Autodesk Fusion 360 part; units mm, degrees
note: some values were not read from the file. Set by a fixed rule: which face or edge a step refers to.
(part 2 of 2)
sketch "Sketch7" plane through (71, 0, 0) normal (1, 0, 0) x (0, 1, 0)
  line L0 (-31, -12) -> (369, -12)
  line L1 (369, -12) -> (348.4062, 44.7862)
  line L2 (348.4062, 44.7862) -> (327.7275, 73.6318)
  line L3 (327.7275, 73.6318) -> (172.6327, 98)
  line L4 (172.6327, 98) -> (-31, 98)
  line L5 (-31, 98) -> (-31, -12)
  line L6 (324.7064, 35.6875) -> (319.5665, 44.4255)
  arc A0 (328.6078, 48.7783) -> (319.5665, 44.4255) centre (321.9697, 51) ccw
  line L7 (328.6078, 48.7783) -> (333.3258, 40.7577)
  arc A1 (338.2936, 32.3125) -> (333.3258, 40.7577) centre (331.5, 34) ccw
  line L8 (338.2936, 32.3125) -> (343.3258, 23.7577)
  arc A2 (348.3189, 15.4181) -> (343.3258, 23.7577) centre (341.5, 17) ccw
  line L9 (348.3189, 15.4181) -> (353.8077, 6.4122)
  arc A3 (346.101, -5) -> (353.8077, 6.4122) centre (351, 0) ccw
  line L10 (346.101, -5) -> (336.399, -5)
  arc A4 (326.601, -5) -> (336.399, -5) centre (331.5, 0) ccw
  line L11 (326.601, -5) -> (316.899, -5)
  arc A5 (310.0903, 6.7345) -> (316.899, -5) centre (312, 0) ccw
  line L12 (310.0903, 6.7345) -> (315.1571, 15.5255)
  arc A6 (319.8454, 23.6602) -> (315.1571, 15.5255) centre (322, 17) ccw
  line L13 (319.8454, 23.6602) -> (324.7456, 32.1622)
  arc A7 (324.7064, 35.6875) -> (324.7456, 32.1622) centre (331.5, 34) ccw
  line L14 (66.4689, 57.708) -> (71.277, 66.0503)
  arc A8 (76.3168, 74.7946) -> (71.277, 66.0503) centre (78, 68) ccw
  line L15 (76.3168, 74.7946) -> (81.1914, 83.2523)
  arc A9 (89.8554, 78.2588) -> (81.1914, 83.2523) centre (87.9697, 85) ccw
  line L16 (89.8554, 78.2588) -> (84.829, 69.5378)
  arc A10 (80.0928, 61.3202) -> (84.829, 69.5378) centre (78, 68) ccw
  line L17 (80.0928, 61.3202) -> (75.2176, 52.8615)
  arc A11 (75.1078, 48.7783) -> (75.2176, 52.8615) centre (68.4697, 51) ccw
  line L18 (75.1078, 48.7783) -> (79.8258, 40.7577)
  arc A12 (84.7936, 32.3125) -> (79.8258, 40.7577) centre (78, 34) ccw
  line L19 (84.7936, 32.3125) -> (89.8258, 23.7577)
  arc A13 (89.6246, 10.1911) -> (89.8258, 23.7577) centre (88, 17) ccw
  line L20 (89.6246, 10.1911) -> (84.7721, 1.7718)
  arc A14 (71.3471, 2.177) -> (84.7721, 1.7718) centre (78, 0) ccw
  line L21 (71.3471, 2.177) -> (66.6451, 10.2502)
  arc A15 (66.3454, 23.6602) -> (66.6451, 10.2502) centre (68.5, 17) ccw
  line L22 (66.3454, 23.6602) -> (71.2456, 32.1622)
  arc A16 (71.2064, 35.6875) -> (71.2456, 32.1622) centre (78, 34) ccw
  line L23 (71.2064, 35.6875) -> (66.0665, 44.4255)
  arc A17 (66.4689, 57.708) -> (66.0665, 44.4255) centre (68.4697, 51) ccw
  line L24 (32.0797, 69.053) -> (26.3996, 78.7092)
  arc A18 (35.9118, 82.2615) -> (26.3996, 78.7092) centre (29.4697, 85) ccw
  line L25 (35.9118, 82.2615) -> (40.2494, 74.8876)
  arc A19 (41.0928, 61.3202) -> (40.2494, 74.8876) centre (39, 68) ccw
  line L26 (41.0928, 61.3202) -> (36.2176, 52.8615)
  arc A20 (36.1078, 48.7783) -> (36.2176, 52.8615) centre (29.4697, 51) ccw
  line L27 (36.1078, 48.7783) -> (40.8258, 40.7577)
  arc A21 (40.9765, 27.2848) -> (40.8258, 40.7577) centre (39, 34) ccw
  line L28 (40.9765, 27.2848) -> (36.2059, 19.0076)
  arc A22 (36.3189, 15.4181) -> (36.2059, 19.0076) centre (29.5, 17) ccw
  line L29 (36.3189, 15.4181) -> (41.8077, 6.4122)
  arc A23 (32.3471, 2.177) -> (41.8077, 6.4122) centre (39, 0) ccw
  line L30 (32.3471, 2.177) -> (27.6451, 10.2502)
  arc A24 (22.7064, 18.6875) -> (27.6451, 10.2502) centre (29.5, 17) ccw
  line L31 (22.7064, 18.6875) -> (17.6742, 27.2423)
  arc A25 (17.7042, 40.7657) -> (17.6742, 27.2423) centre (19.5, 34) ccw
  line L32 (17.7042, 40.7657) -> (22.6625, 49.3685)
  arc A26 (27.4689, 57.708) -> (22.6625, 49.3685) centre (29.4697, 51) ccw
  line L33 (27.4689, 57.708) -> (32.277, 66.0503)
  arc A27 (32.0797, 69.053) -> (32.277, 66.0503) centre (39, 68) ccw
  line L34 (-1.6832, 74.7946) -> (3.1914, 83.2523)
  arc A28 (16.4118, 82.2615) -> (3.1914, 83.2523) centre (9.9697, 85) ccw
  line L35 (16.4118, 82.2615) -> (20.7494, 74.8876)
  arc A29 (21.5928, 61.3202) -> (20.7494, 74.8876) centre (19.5, 68) ccw
  line L36 (21.5928, 61.3202) -> (16.7176, 52.8615)
  arc A30 (11.7417, 44.228) -> (16.7176, 52.8615) centre (9.9697, 51) ccw
  line L37 (11.7417, 44.228) -> (6.8013, 35.6561)
  arc A31 (6.7936, 32.3125) -> (6.8013, 35.6561) centre (0, 34) ccw
  line L38 (6.7936, 32.3125) -> (11.8258, 23.7577)
  arc A32 (16.8189, 15.4181) -> (11.8258, 23.7577) centre (10, 17) ccw
  line L39 (16.8189, 15.4181) -> (22.3077, 6.4122)
  arc A33 (12.8471, 2.177) -> (22.3077, 6.4122) centre (19.5, 0) ccw
  line L40 (12.8471, 2.177) -> (8.1451, 10.2502)
  arc A34 (3.2064, 18.6875) -> (8.1451, 10.2502) centre (10, 17) ccw
  line L41 (3.2064, 18.6875) -> (-1.8258, 27.2423)
  arc A35 (-1.7958, 40.7657) -> (-1.8258, 27.2423) centre (0, 34) ccw
  line L42 (-1.7958, 40.7657) -> (3.1625, 49.3685)
  arc A36 (3.0557, 52.0938) -> (3.1625, 49.3685) centre (9.9697, 51) ccw
  line L43 (3.0557, 52.0938) -> (-2.4419, 61.4397)
  arc A37 (-1.6832, 74.7946) -> (-2.4419, 61.4397) centre (0, 68) ccw
  line L44 (-21.1832, 74.7946) -> (-16.3086, 83.2523)
  arc A38 (-7.6446, 78.2588) -> (-16.3086, 83.2523) centre (-9.5303, 85) ccw
  line L45 (-7.6446, 78.2588) -> (-12.671, 69.5378)
  arc A39 (-12.873, 65.7456) -> (-12.671, 69.5378) centre (-19.5, 68) ccw
  line L46 (-12.873, 65.7456) -> (-8.2469, 57.8813)
  arc A40 (-7.7583, 44.228) -> (-8.2469, 57.8813) centre (-9.5303, 51) ccw
  line L47 (-7.7583, 44.228) -> (-12.6987, 35.6561)
  arc A41 (-12.7064, 32.3125) -> (-12.6987, 35.6561) centre (-19.5, 34) ccw
  line L48 (-12.7064, 32.3125) -> (-7.6742, 23.7577)
  arc A42 (-2.6811, 15.4181) -> (-7.6742, 23.7577) centre (-9.5, 17) ccw
  line L49 (-2.6811, 15.4181) -> (2.8077, 6.4122)
  arc A43 (-4.899, -5) -> (2.8077, 6.4122) centre (0, 0) ccw
  line L50 (-4.899, -5) -> (-14.601, -5)
  arc A44 (-21.4097, 6.7345) -> (-14.601, -5) centre (-19.5, 0) ccw
  line L51 (-21.4097, 6.7345) -> (-16.3429, 15.5255)
  arc A45 (-16.2936, 18.6875) -> (-16.3429, 15.5255) centre (-9.5, 17) ccw
  line L52 (-16.2936, 18.6875) -> (-21.3258, 27.2423)
  arc A46 (-21.2958, 40.7657) -> (-21.3258, 27.2423) centre (-19.5, 34) ccw
  line L53 (-21.2958, 40.7657) -> (-16.3375, 49.3685)
  arc A47 (-16.4443, 52.0938) -> (-16.3375, 49.3685) centre (-9.5303, 51) ccw
  line L54 (-16.4443, 52.0938) -> (-21.9419, 61.4397)
  arc A48 (-21.1832, 74.7946) -> (-21.9419, 61.4397) centre (-19.5, 68) ccw
  line L55 (193.3168, 74.7946) -> (194.7952, 77.3597)
  line L56 (194.7952, 77.3597) -> (196.2494, 74.8876)
  arc A49 (201.627, 65.7456) -> (196.2494, 74.8876) centre (195, 68) ccw
  line L57 (201.627, 65.7456) -> (206.2531, 57.8813)
  arc A50 (206.7417, 44.228) -> (206.2531, 57.8813) centre (204.9697, 51) ccw
  line L58 (206.7417, 44.228) -> (201.8013, 35.6561)
  arc A51 (201.7936, 32.3125) -> (201.8013, 35.6561) centre (195, 34) ccw
  line L59 (201.7936, 32.3125) -> (206.8258, 23.7577)
  arc A52 (206.6246, 10.1911) -> (206.8258, 23.7577) centre (205, 17) ccw
  line L60 (206.6246, 10.1911) -> (201.7721, 1.7718)
  arc A53 (188.3471, 2.177) -> (201.7721, 1.7718) centre (195, 0) ccw
  line L61 (188.3471, 2.177) -> (183.6451, 10.2502)
  arc A54 (183.3454, 23.6602) -> (183.6451, 10.2502) centre (185.5, 17) ccw
  line L62 (183.3454, 23.6602) -> (188.2456, 32.1622)
  arc A55 (188.2064, 35.6875) -> (188.2456, 32.1622) centre (195, 34) ccw
  line L63 (188.2064, 35.6875) -> (183.0665, 44.4255)
  arc A56 (183.4689, 57.708) -> (183.0665, 44.4255) centre (185.4697, 51) ccw
  line L64 (183.4689, 57.708) -> (188.277, 66.0503)
  arc A57 (193.3168, 74.7946) -> (188.277, 66.0503) centre (195, 68) ccw
  line L65 (55.8189, 15.4181) -> (61.3077, 6.4122)
  arc A58 (51.8471, 2.177) -> (61.3077, 6.4122) centre (58.5, 0) ccw
  line L66 (51.8471, 2.177) -> (47.1451, 10.2502)
  arc A59 (46.8454, 23.6602) -> (47.1451, 10.2502) centre (49, 17) ccw
  line L67 (46.8454, 23.6602) -> (51.7456, 32.1622)
  arc A60 (51.7064, 35.6875) -> (51.7456, 32.1622) centre (58.5, 34) ccw
  line L68 (51.7064, 35.6875) -> (46.5665, 44.4255)
  arc A61 (46.9689, 57.708) -> (46.5665, 44.4255) centre (48.9697, 51) ccw
  line L69 (46.9689, 57.708) -> (51.777, 66.0503)
  arc A62 (51.5797, 69.053) -> (51.777, 66.0503) centre (58.5, 68) ccw
  line L70 (51.5797, 69.053) -> (45.8996, 78.7092)
  arc A63 (53.8686, 90) -> (45.8996, 78.7092) centre (48.9697, 85) ccw
  line L71 (53.8686, 90) -> (63.5707, 90)
  arc A64 (70.3554, 78.2588) -> (63.5707, 90) centre (68.4697, 85) ccw
  line L72 (70.3554, 78.2588) -> (65.329, 69.5378)
  arc A65 (60.5928, 61.3202) -> (65.329, 69.5378) centre (58.5, 68) ccw
  line L73 (60.5928, 61.3202) -> (55.7176, 52.8615)
  arc A66 (55.6078, 48.7783) -> (55.7176, 52.8615) centre (48.9697, 51) ccw
  line L74 (55.6078, 48.7783) -> (60.3258, 40.7577)
  arc A67 (60.4765, 27.2848) -> (60.3258, 40.7577) centre (58.5, 34) ccw
  line L75 (60.4765, 27.2848) -> (55.7059, 19.0076)
  arc A68 (55.8189, 15.4181) -> (55.7059, 19.0076) centre (49, 17) ccw
  line L76 (95.8168, 74.7946) -> (100.6914, 83.2523)
  arc A69 (109.3554, 78.2588) -> (100.6914, 83.2523) centre (107.4697, 85) ccw
  line L77 (109.3554, 78.2588) -> (104.329, 69.5378)
  arc A70 (104.127, 65.7456) -> (104.329, 69.5378) centre (97.5, 68) ccw
  line L78 (104.127, 65.7456) -> (108.7531, 57.8813)
  arc A71 (109.2417, 44.228) -> (108.7531, 57.8813) centre (107.4697, 51) ccw
  line L79 (109.2417, 44.228) -> (104.3013, 35.6561)
  arc A72 (104.2936, 32.3125) -> (104.3013, 35.6561) centre (97.5, 34) ccw
  line L80 (104.2936, 32.3125) -> (109.3258, 23.7577)
  arc A73 (109.1246, 10.1911) -> (109.3258, 23.7577) centre (107.5, 17) ccw
  line L81 (109.1246, 10.1911) -> (104.2721, 1.7718)
  arc A74 (95.5903, 6.7345) -> (104.2721, 1.7718) centre (97.5, 0) ccw
  line L82 (95.5903, 6.7345) -> (100.6571, 15.5255)
  arc A75 (100.7064, 18.6875) -> (100.6571, 15.5255) centre (107.5, 17) ccw
  line L83 (100.7064, 18.6875) -> (95.6742, 27.2423)
  arc A76 (90.7064, 35.6875) -> (95.6742, 27.2423) centre (97.5, 34) ccw
  line L84 (90.7064, 35.6875) -> (85.5665, 44.4255)
  arc A77 (85.9689, 57.708) -> (85.5665, 44.4255) centre (87.9697, 51) ccw
  line L85 (85.9689, 57.708) -> (90.777, 66.0503)
  arc A78 (95.8168, 74.7946) -> (90.777, 66.0503) centre (97.5, 68) ccw
  line L86 (268.101, -5) -> (258.399, -5)
  arc A79 (251.5903, 6.7345) -> (258.399, -5) centre (253.5, 0) ccw
  line L87 (251.5903, 6.7345) -> (256.6571, 15.5255)
  arc A80 (256.7064, 18.6875) -> (256.6571, 15.5255) centre (263.5, 17) ccw
  line L88 (256.7064, 18.6875) -> (251.6742, 27.2423)
  arc A81 (246.7064, 35.6875) -> (251.6742, 27.2423) centre (253.5, 34) ccw
  line L89 (246.7064, 35.6875) -> (241.5665, 44.4255)
  arc A82 (248.8686, 56) -> (241.5665, 44.4255) centre (243.9697, 51) ccw
  line L90 (248.8686, 56) -> (258.5707, 56)
  arc A83 (270.1078, 48.7783) -> (258.5707, 56) centre (263.4697, 51) ccw
  line L91 (270.1078, 48.7783) -> (274.8258, 40.7577)
  arc A84 (274.9765, 27.2848) -> (274.8258, 40.7577) centre (273, 34) ccw
  line L92 (274.9765, 27.2848) -> (270.2059, 19.0076)
  arc A85 (270.3189, 15.4181) -> (270.2059, 19.0076) centre (263.5, 17) ccw
  line L93 (270.3189, 15.4181) -> (275.8077, 6.4122)
  arc A86 (268.101, -5) -> (275.8077, 6.4122) centre (273, 0) ccw
  line L94 (134.8168, 74.7946) -> (139.6914, 83.2523)
  arc A87 (148.3554, 78.2588) -> (139.6914, 83.2523) centre (146.4697, 85) ccw
  line L95 (148.3554, 78.2588) -> (143.329, 69.5378)
  arc A88 (143.127, 65.7456) -> (143.329, 69.5378) centre (136.5, 68) ccw
  line L96 (143.127, 65.7456) -> (147.7531, 57.8813)
  arc A89 (153.1078, 48.7783) -> (147.7531, 57.8813) centre (146.4697, 51) ccw
  line L97 (153.1078, 48.7783) -> (157.8258, 40.7577)
  arc A90 (157.9765, 27.2848) -> (157.8258, 40.7577) centre (156, 34) ccw
  line L98 (157.9765, 27.2848) -> (153.2059, 19.0076)
  arc A91 (153.3189, 15.4181) -> (153.2059, 19.0076) centre (146.5, 17) ccw
  line L99 (153.3189, 15.4181) -> (158.8077, 6.4122)
  arc A92 (149.3471, 2.177) -> (158.8077, 6.4122) centre (156, 0) ccw
  line L100 (149.3471, 2.177) -> (144.6451, 10.2502)
  arc A93 (139.7064, 18.6875) -> (144.6451, 10.2502) centre (146.5, 17) ccw
  line L101 (139.7064, 18.6875) -> (134.6742, 27.2423)
  arc A94 (134.7042, 40.7657) -> (134.6742, 27.2423) centre (136.5, 34) ccw
  line L102 (134.7042, 40.7657) -> (139.6625, 49.3685)
  arc A95 (139.5557, 52.0938) -> (139.6625, 49.3685) centre (146.4697, 51) ccw
  line L103 (139.5557, 52.0938) -> (134.0581, 61.4397)
  arc A96 (134.8168, 74.7946) -> (134.0581, 61.4397) centre (136.5, 68) ccw
  line L104 (280.8454, 23.6602) -> (285.7456, 32.1622)
  arc A97 (285.7064, 35.6875) -> (285.7456, 32.1622) centre (292.5, 34) ccw
  line L105 (285.7064, 35.6875) -> (280.5665, 44.4255)
  arc A98 (287.8686, 56) -> (280.5665, 44.4255) centre (282.9697, 51) ccw
  line L106 (287.8686, 56) -> (297.5707, 56)
  arc A99 (309.1078, 48.7783) -> (297.5707, 56) centre (302.4697, 51) ccw
  line L107 (309.1078, 48.7783) -> (313.8258, 40.7577)
  arc A100 (313.9765, 27.2848) -> (313.8258, 40.7577) centre (312, 34) ccw
  line L108 (313.9765, 27.2848) -> (309.2059, 19.0076)
  arc A101 (304.1246, 10.1911) -> (309.2059, 19.0076) centre (302.5, 17) ccw
  line L109 (304.1246, 10.1911) -> (299.2721, 1.7718)
  arc A102 (285.8471, 2.177) -> (299.2721, 1.7718) centre (292.5, 0) ccw
  line L110 (285.8471, 2.177) -> (281.1451, 10.2502)
  arc A103 (280.8454, 23.6602) -> (281.1451, 10.2502) centre (283, 17) ccw
  line L111 (172.8189, 15.4181) -> (178.3077, 6.4122)
  arc A104 (168.8471, 2.177) -> (178.3077, 6.4122) centre (175.5, 0) ccw
  line L112 (168.8471, 2.177) -> (164.1451, 10.2502)
  arc A105 (163.8454, 23.6602) -> (164.1451, 10.2502) centre (166, 17) ccw
  line L113 (163.8454, 23.6602) -> (168.7456, 32.1622)
  arc A106 (168.7064, 35.6875) -> (168.7456, 32.1622) centre (175.5, 34) ccw
  line L114 (168.7064, 35.6875) -> (163.5665, 44.4255)
  arc A107 (159.0557, 52.0938) -> (163.5665, 44.4255) centre (165.9697, 51) ccw
  line L115 (159.0557, 52.0938) -> (153.5581, 61.4397)
  arc A108 (154.3168, 74.7946) -> (153.5581, 61.4397) centre (156, 68) ccw
  line L116 (154.3168, 74.7946) -> (159.1914, 83.2523)
  arc A109 (172.4118, 82.2615) -> (159.1914, 83.2523) centre (165.9697, 85) ccw
  line L117 (172.4118, 82.2615) -> (176.7494, 74.8876)
  arc A110 (177.5928, 61.3202) -> (176.7494, 74.8876) centre (175.5, 68) ccw
  line L118 (177.5928, 61.3202) -> (172.7176, 52.8615)
  arc A111 (172.6078, 48.7783) -> (172.7176, 52.8615) centre (165.9697, 51) ccw
  line L119 (172.6078, 48.7783) -> (177.3258, 40.7577)
  arc A112 (177.4765, 27.2848) -> (177.3258, 40.7577) centre (175.5, 34) ccw
  line L120 (177.4765, 27.2848) -> (172.7059, 19.0076)
  arc A113 (172.8189, 15.4181) -> (172.7059, 19.0076) centre (166, 17) ccw
  line L121 (115.3168, 74.7946) -> (120.1914, 83.2523)
  arc A114 (128.8554, 78.2588) -> (120.1914, 83.2523) centre (126.9697, 85) ccw
  line L122 (128.8554, 78.2588) -> (123.829, 69.5378)
  arc A115 (123.627, 65.7456) -> (123.829, 69.5378) centre (117, 68) ccw
  line L123 (123.627, 65.7456) -> (128.2531, 57.8813)
  arc A116 (128.7417, 44.228) -> (128.2531, 57.8813) centre (126.9697, 51) ccw
  line L124 (128.7417, 44.228) -> (123.8013, 35.6561)
  arc A117 (123.7936, 32.3125) -> (123.8013, 35.6561) centre (117, 34) ccw
  line L125 (123.7936, 32.3125) -> (128.8258, 23.7577)
  arc A118 (133.8189, 15.4181) -> (128.8258, 23.7577) centre (127, 17) ccw
  line L126 (133.8189, 15.4181) -> (139.3077, 6.4122)
  arc A119 (131.601, -5) -> (139.3077, 6.4122) centre (136.5, 0) ccw
  line L127 (131.601, -5) -> (121.899, -5)
  arc A120 (115.0903, 6.7345) -> (121.899, -5) centre (117, 0) ccw
  line L128 (115.0903, 6.7345) -> (120.1571, 15.5255)
  arc A121 (120.2064, 18.6875) -> (120.1571, 15.5255) centre (127, 17) ccw
  line L129 (120.2064, 18.6875) -> (115.1742, 27.2423)
  arc A122 (115.2042, 40.7657) -> (115.1742, 27.2423) centre (117, 34) ccw
  line L130 (115.2042, 40.7657) -> (120.1625, 49.3685)
  arc A123 (120.0557, 52.0938) -> (120.1625, 49.3685) centre (126.9697, 51) ccw
  line L131 (120.0557, 52.0938) -> (114.5581, 61.4397)
  arc A124 (115.3168, 74.7946) -> (114.5581, 61.4397) centre (117, 68) ccw
  line L132 (212.7042, 40.7657) -> (217.6625, 49.3685)
  arc A125 (231.1078, 48.7783) -> (217.6625, 49.3685) centre (224.4697, 51) ccw
  line L133 (231.1078, 48.7783) -> (235.8258, 40.7577)
  arc A126 (240.7936, 32.3125) -> (235.8258, 40.7577) centre (234, 34) ccw
  line L134 (240.7936, 32.3125) -> (245.8258, 23.7577)
  arc A127 (245.6246, 10.1911) -> (245.8258, 23.7577) centre (244, 17) ccw
  line L135 (245.6246, 10.1911) -> (240.7721, 1.7718)
  arc A128 (229.101, -5) -> (240.7721, 1.7718) centre (234, 0) ccw
  line L136 (229.101, -5) -> (219.399, -5)
  arc A129 (212.5903, 6.7345) -> (219.399, -5) centre (214.5, 0) ccw
  line L137 (212.5903, 6.7345) -> (217.6571, 15.5255)
  arc A130 (217.7064, 18.6875) -> (217.6571, 15.5255) centre (224.5, 17) ccw
  line L138 (217.7064, 18.6875) -> (212.6742, 27.2423)
  arc A131 (212.7042, 40.7657) -> (212.6742, 27.2423) centre (214.5, 34) ccw
  line L139 (-9.5303, 85) -> (165.9697, 85) construction
  line L140 (-18.3947, 90) -> (350, 90)
  line L141 (-45, 80) -> (350, 80)
  line L142 (-45, 63) -> (350, 63)
  line L143 (-18.3947, 73) -> (350, 73)
  line L144 (-45, 46) -> (350, 46)
  line L145 (-18.3947, 56) -> (350, 56)
  line L146 (-45, 29) -> (350, 29)
  line L147 (-18.3947, 39) -> (350, 39)
  line L148 (-45, 12) -> (350, 12)
  line L149 (-18.3947, 22) -> (350, 22)
  line L150 (-45, -5) -> (350, -5)
  line L151 (-18.3947, 5) -> (350, 5)
  line L152 (-12.0046, 90) -> (-12.0046, 102)
  line L153 (-7.9736, 90) -> (-7.9736, 102)
  line L154 (-12.0046, 96) -> (-7.9736, 96)
  line L155 (321.9697, 58) -> (317.9396, 75.1697)
  line L156 (317.0707, 56) -> (312.3656, 76.0454)
  line L157 (313.4417, 71.4611) -> (318.8101, 71.4611)
  dimension "d339" = 5
  dimension "d340" = 5
  dimension "d343" = 0
  dimension "d344" = -17
  constraint coincident A38.centre L139.start
  constraint coincident A109.centre L139.end
  constraint parallel L4 L140
  constraint horizontal L141
  constraint coincident L140 L152.start
  constraint perpendicular L140 L152
  constraint coincident L140 L153.start
  constraint perpendicular L4 L153
  constraint midpoint L152 L154.start
  constraint midpoint L153 L154.end
  constraint perpendicular L153 L154
  constraint coincident A0 L155.start
  constraint coincident L3 L155.end
  constraint coincident A0 L156.start
  constraint coincident L145 L156.start
  constraint coincident L3 L156.end
  constraint parallel L155 L156
  constraint coincident L156 L157.start
  constraint coincident L155 L157.end
  constraint parallel L143 L157
  measures "d339" distance of L139 L140
  measures "d340" distance of A9.centre L141
extrude "Extrude16" cut sketch "Sketch7" against normal blind 2.2 contours L30 A24 L39 A33 L148 L151 | A24 L31 A32 L39 L148 L149 | A83 L91 A98 L144 L145 | L91 A84 L105 A98 L144 L147 | L31 A25 L38 A32 L146 L149 | A25 L37 A31 L38 L146 L147 | A23 L30 A33 L150 L151 | A25 L32 A30 L37 L144 L147 | L32 A26 L36 A30 L144 L145 | A84 L104 A97 L105 L146 L147 | A26 L33 A29 L36 L142 L145 | L24 L33 A27 A29 L142 L143 | A50 L132 A125 L144 L145 | A84 L92 L104 A103 L146 L149 | L24 A18 L35 A29 L141 L143 | A18 A28 L35 L140 L141 | L21 A15 L65 A58 L148 L151 | A15 L65 L75 A68 L148 L149 | A50 L58 L132 A131 L144 L147 | L95 A88 L96 A108 L142 L143 | L96 A89 L115 A108 L142 L145 | A15 L22 A67 L75 L146 L149 | L22 A16 L23 A67 L146 L147 | A14 L21 A58 L150 L151 | A87 L116 A109 L140 L141 | A87 L95 A108 L116 L141 L143 | L92 A85 L93 A103 L148 L149 | L23 A17 L74 A67 L144 L147 | A17 L73 A66 L74 L144 L145 | L58 A51 L59 A131 L146 L147 | A89 L97 A107 L115 L144 L145 | L93 A86 L110 A103 L148 L151 | L14 A17 A65 L73 L142 L145 | L14 A8 L72 A65 L142 L143 | L97 A90 L114 A107 L144 L147 | L59 A52 L138 A131 L146 L149 | A8 L15 A64 L72 L141 L143 | L15 A9 A64 L140 L141 | A73 L81 A120 L128 L148 L151 | A73 L128 A121 L129 L148 L149 | L77 A70 L78 A124 L142 L143 | L78 A71 L131 A124 L142 L145 | A86 A102 L110 L150 L151 | L80 A73 L129 A122 L146 L149 | L79 A72 L80 A122 L146 L147 | L81 A74 A120 L150 L151 | A69 L121 A114 L140 L141 | A69 L77 L121 A124 L141 L143 | A90 L113 A106 L114 L146 L147 | A52 L137 A130 L138 L148 L149 | A71 L79 A122 L130 L144 L147 | A71 L130 A123 L131 L144 L145 | A90 L98 A105 L113 L146 L149 | A52 L60 A129 L137 L148 L151 | L99 A92 L112 A105 L148 L151 | L98 A91 L99 A105 L148 L149 | L60 A53 A129 L150 L151 | A92 A104 L112 L150 L151 bodies 3
sketch "Sketch8" plane through (0, 0, 0) normal (-1, 0, 0) x (0, -1, 0)
  line L0 (-369, -12) -> (31, -12)
  line L1 (31, -12) -> (31, 98)
  line L2 (31, 98) -> (-172.6327, 98)
  line L3 (-172.6327, 98) -> (-327.7275, 73.6318)
  line L4 (-327.7275, 73.6318) -> (-348.4062, 44.7862)
  line L5 (-348.4062, 44.7862) -> (-369, -12)
  line L6 (-319.5665, 44.4255) -> (-324.7064, 35.6875)
  arc A0 (-324.7456, 32.1622) -> (-324.7064, 35.6875) centre (-331.5, 34) ccw
  line L7 (-324.7456, 32.1622) -> (-319.8454, 23.6602)
  arc A1 (-315.1571, 15.5255) -> (-319.8454, 23.6602) centre (-322, 17) ccw
  line L8 (-315.1571, 15.5255) -> (-310.0903, 6.7345)
  arc A2 (-316.899, -5) -> (-310.0903, 6.7345) centre (-312, 0) ccw
  line L9 (-316.899, -5) -> (-326.601, -5)
  arc A3 (-336.399, -5) -> (-326.601, -5) centre (-331.5, 0) ccw
  line L10 (-336.399, -5) -> (-346.101, -5)
  arc A4 (-353.8077, 6.4122) -> (-346.101, -5) centre (-351, 0) ccw
  line L11 (-353.8077, 6.4122) -> (-348.3189, 15.4181)
  arc A5 (-343.3258, 23.7577) -> (-348.3189, 15.4181) centre (-341.5, 17) ccw
  line L12 (-343.3258, 23.7577) -> (-338.2936, 32.3125)
  arc A6 (-333.3258, 40.7577) -> (-338.2936, 32.3125) centre (-331.5, 34) ccw
  line L13 (-333.3258, 40.7577) -> (-328.6078, 48.7783)
  arc A7 (-319.5665, 44.4255) -> (-328.6078, 48.7783) centre (-321.9697, 51) ccw
  line L14 (-71.277, 66.0503) -> (-66.4689, 57.708)
  arc A8 (-66.0665, 44.4255) -> (-66.4689, 57.708) centre (-68.4697, 51) ccw
  line L15 (-66.0665, 44.4255) -> (-71.2064, 35.6875)
  arc A9 (-71.2456, 32.1622) -> (-71.2064, 35.6875) centre (-78, 34) ccw
  line L16 (-71.2456, 32.1622) -> (-66.3454, 23.6602)
  arc A10 (-66.6451, 10.2502) -> (-66.3454, 23.6602) centre (-68.5, 17) ccw
  line L17 (-66.6451, 10.2502) -> (-71.3471, 2.177)
  arc A11 (-84.7721, 1.7718) -> (-71.3471, 2.177) centre (-78, 0) ccw
  line L18 (-84.7721, 1.7718) -> (-89.6246, 10.1911)
  arc A12 (-89.8258, 23.7577) -> (-89.6246, 10.1911) centre (-88, 17) ccw
  line L19 (-89.8258, 23.7577) -> (-84.7936, 32.3125)
  arc A13 (-79.8258, 40.7577) -> (-84.7936, 32.3125) centre (-78, 34) ccw
  line L20 (-79.8258, 40.7577) -> (-75.1078, 48.7783)
  arc A14 (-75.2176, 52.8615) -> (-75.1078, 48.7783) centre (-68.4697, 51) ccw
  line L21 (-75.2176, 52.8615) -> (-80.0928, 61.3202)
  arc A15 (-84.829, 69.5378) -> (-80.0928, 61.3202) centre (-78, 68) ccw
  line L22 (-84.829, 69.5378) -> (-89.8554, 78.2588)
  arc A16 (-81.1914, 83.2523) -> (-89.8554, 78.2588) centre (-87.9697, 85) ccw
  line L23 (-81.1914, 83.2523) -> (-76.3168, 74.7946)
  arc A17 (-71.277, 66.0503) -> (-76.3168, 74.7946) centre (-78, 68) ccw
  line L24 (-26.3996, 78.7092) -> (-32.0797, 69.053)
  arc A18 (-32.277, 66.0503) -> (-32.0797, 69.053) centre (-39, 68) ccw
  line L25 (-32.277, 66.0503) -> (-27.4689, 57.708)
  arc A19 (-22.6625, 49.3685) -> (-27.4689, 57.708) centre (-29.4697, 51) ccw
  line L26 (-22.6625, 49.3685) -> (-17.7042, 40.7657)
  arc A20 (-17.6742, 27.2423) -> (-17.7042, 40.7657) centre (-19.5, 34) ccw
  line L27 (-17.6742, 27.2423) -> (-22.7064, 18.6875)
  arc A21 (-27.6451, 10.2502) -> (-22.7064, 18.6875) centre (-29.5, 17) ccw
  line L28 (-27.6451, 10.2502) -> (-32.3471, 2.177)
  arc A22 (-41.8077, 6.4122) -> (-32.3471, 2.177) centre (-39, 0) ccw
  line L29 (-41.8077, 6.4122) -> (-36.3189, 15.4181)
  arc A23 (-36.2059, 19.0076) -> (-36.3189, 15.4181) centre (-29.5, 17) ccw
  line L30 (-36.2059, 19.0076) -> (-40.9765, 27.2848)
  arc A24 (-40.8258, 40.7577) -> (-40.9765, 27.2848) centre (-39, 34) ccw
  line L31 (-40.8258, 40.7577) -> (-36.1078, 48.7783)
  arc A25 (-36.2176, 52.8615) -> (-36.1078, 48.7783) centre (-29.4697, 51) ccw
  line L32 (-36.2176, 52.8615) -> (-41.0928, 61.3202)
  arc A26 (-40.2494, 74.8876) -> (-41.0928, 61.3202) centre (-39, 68) ccw
  line L33 (-40.2494, 74.8876) -> (-35.9118, 82.2615)
  arc A27 (-26.3996, 78.7092) -> (-35.9118, 82.2615) centre (-29.4697, 85) ccw
  line L34 (-3.1914, 83.2523) -> (1.6832, 74.7946)
  arc A28 (2.4419, 61.4397) -> (1.6832, 74.7946) centre (0, 68) ccw
  line L35 (2.4419, 61.4397) -> (-3.0557, 52.0938)
  arc A29 (-3.1625, 49.3685) -> (-3.0557, 52.0938) centre (-9.9697, 51) ccw
  line L36 (-3.1625, 49.3685) -> (1.7958, 40.7657)
  arc A30 (1.8258, 27.2423) -> (1.7958, 40.7657) centre (0, 34) ccw
  line L37 (1.8258, 27.2423) -> (-3.2064, 18.6875)
  arc A31 (-8.1451, 10.2502) -> (-3.2064, 18.6875) centre (-10, 17) ccw
  line L38 (-8.1451, 10.2502) -> (-12.8471, 2.177)
  arc A32 (-22.3077, 6.4122) -> (-12.8471, 2.177) centre (-19.5, 0) ccw
  line L39 (-22.3077, 6.4122) -> (-16.8189, 15.4181)
  arc A33 (-11.8258, 23.7577) -> (-16.8189, 15.4181) centre (-10, 17) ccw
  line L40 (-11.8258, 23.7577) -> (-6.7936, 32.3125)
  arc A34 (-6.8013, 35.6561) -> (-6.7936, 32.3125) centre (0, 34) ccw
  line L41 (-6.8013, 35.6561) -> (-11.7417, 44.228)
  arc A35 (-16.7176, 52.8615) -> (-11.7417, 44.228) centre (-9.9697, 51) ccw
  line L42 (-16.7176, 52.8615) -> (-21.5928, 61.3202)
  arc A36 (-20.7494, 74.8876) -> (-21.5928, 61.3202) centre (-19.5, 68) ccw
  line L43 (-20.7494, 74.8876) -> (-16.4118, 82.2615)
  arc A37 (-3.1914, 83.2523) -> (-16.4118, 82.2615) centre (-9.9697, 85) ccw
  line L44 (16.3086, 83.2523) -> (21.1832, 74.7946)
  arc A38 (21.9419, 61.4397) -> (21.1832, 74.7946) centre (19.5, 68) ccw
  line L45 (21.9419, 61.4397) -> (16.4443, 52.0938)
  arc A39 (16.3375, 49.3685) -> (16.4443, 52.0938) centre (9.5303, 51) ccw
  line L46 (16.3375, 49.3685) -> (21.2958, 40.7657)
  arc A40 (21.3258, 27.2423) -> (21.2958, 40.7657) centre (19.5, 34) ccw
  line L47 (21.3258, 27.2423) -> (16.2936, 18.6875)
  arc A41 (16.3429, 15.5255) -> (16.2936, 18.6875) centre (9.5, 17) ccw
  line L48 (16.3429, 15.5255) -> (21.4097, 6.7345)
  arc A42 (14.601, -5) -> (21.4097, 6.7345) centre (19.5, 0) ccw
  line L49 (14.601, -5) -> (4.899, -5)
  arc A43 (-2.8077, 6.4122) -> (4.899, -5) centre (0, 0) ccw
  line L50 (-2.8077, 6.4122) -> (2.6811, 15.4181)
  arc A44 (7.6742, 23.7577) -> (2.6811, 15.4181) centre (9.5, 17) ccw
  line L51 (7.6742, 23.7577) -> (12.7064, 32.3125)
  arc A45 (12.6987, 35.6561) -> (12.7064, 32.3125) centre (19.5, 34) ccw
  line L52 (12.6987, 35.6561) -> (7.7583, 44.228)
  arc A46 (8.2469, 57.8813) -> (7.7583, 44.228) centre (9.5303, 51) ccw
  line L53 (8.2469, 57.8813) -> (12.873, 65.7456)
  arc A47 (12.671, 69.5378) -> (12.873, 65.7456) centre (19.5, 68) ccw
  line L54 (12.671, 69.5378) -> (7.6446, 78.2588)
  arc A48 (16.3086, 83.2523) -> (7.6446, 78.2588) centre (9.5303, 85) ccw
  line L55 (-194.7952, 77.3597) -> (-193.3168, 74.7946)
  arc A49 (-188.277, 66.0503) -> (-193.3168, 74.7946) centre (-195, 68) ccw
  line L56 (-188.277, 66.0503) -> (-183.4689, 57.708)
  arc A50 (-183.0665, 44.4255) -> (-183.4689, 57.708) centre (-185.4697, 51) ccw
  line L57 (-183.0665, 44.4255) -> (-188.2064, 35.6875)
  arc A51 (-188.2456, 32.1622) -> (-188.2064, 35.6875) centre (-195, 34) ccw
  line L58 (-188.2456, 32.1622) -> (-183.3454, 23.6602)
  arc A52 (-183.6451, 10.2502) -> (-183.3454, 23.6602) centre (-185.5, 17) ccw
  line L59 (-183.6451, 10.2502) -> (-188.3471, 2.177)
  arc A53 (-201.7721, 1.7718) -> (-188.3471, 2.177) centre (-195, 0) ccw
  line L60 (-201.7721, 1.7718) -> (-206.6246, 10.1911)
  arc A54 (-206.8258, 23.7577) -> (-206.6246, 10.1911) centre (-205, 17) ccw
  line L61 (-206.8258, 23.7577) -> (-201.7936, 32.3125)
  arc A55 (-201.8013, 35.6561) -> (-201.7936, 32.3125) centre (-195, 34) ccw
  line L62 (-201.8013, 35.6561) -> (-206.7417, 44.228)
  arc A56 (-206.2531, 57.8813) -> (-206.7417, 44.228) centre (-204.9697, 51) ccw
  line L63 (-206.2531, 57.8813) -> (-201.627, 65.7456)
  arc A57 (-196.2494, 74.8876) -> (-201.627, 65.7456) centre (-195, 68) ccw
  line L64 (-196.2494, 74.8876) -> (-194.7952, 77.3597)
  line L65 (-61.3077, 6.4122) -> (-55.8189, 15.4181)
  arc A58 (-55.7059, 19.0076) -> (-55.8189, 15.4181) centre (-49, 17) ccw
  line L66 (-55.7059, 19.0076) -> (-60.4765, 27.2848)
  arc A59 (-60.3258, 40.7577) -> (-60.4765, 27.2848) centre (-58.5, 34) ccw
  line L67 (-60.3258, 40.7577) -> (-55.6078, 48.7783)
  arc A60 (-55.7176, 52.8615) -> (-55.6078, 48.7783) centre (-48.9697, 51) ccw
  line L68 (-55.7176, 52.8615) -> (-60.5928, 61.3202)
  arc A61 (-65.329, 69.5378) -> (-60.5928, 61.3202) centre (-58.5, 68) ccw
  line L69 (-65.329, 69.5378) -> (-70.3554, 78.2588)
  arc A62 (-63.5707, 90) -> (-70.3554, 78.2588) centre (-68.4697, 85) ccw
  line L70 (-63.5707, 90) -> (-53.8686, 90)
  arc A63 (-45.8996, 78.7092) -> (-53.8686, 90) centre (-48.9697, 85) ccw
  line L71 (-45.8996, 78.7092) -> (-51.5797, 69.053)
  arc A64 (-51.777, 66.0503) -> (-51.5797, 69.053) centre (-58.5, 68) ccw
  line L72 (-51.777, 66.0503) -> (-46.9689, 57.708)
  arc A65 (-46.5665, 44.4255) -> (-46.9689, 57.708) centre (-48.9697, 51) ccw
  line L73 (-46.5665, 44.4255) -> (-51.7064, 35.6875)
  arc A66 (-51.7456, 32.1622) -> (-51.7064, 35.6875) centre (-58.5, 34) ccw
  line L74 (-51.7456, 32.1622) -> (-46.8454, 23.6602)
  arc A67 (-47.1451, 10.2502) -> (-46.8454, 23.6602) centre (-49, 17) ccw
  line L75 (-47.1451, 10.2502) -> (-51.8471, 2.177)
  arc A68 (-61.3077, 6.4122) -> (-51.8471, 2.177) centre (-58.5, 0) ccw
  line L76 (-100.6914, 83.2523) -> (-95.8168, 74.7946)
  arc A69 (-90.777, 66.0503) -> (-95.8168, 74.7946) centre (-97.5, 68) ccw
  line L77 (-90.777, 66.0503) -> (-85.9689, 57.708)
  arc A70 (-85.5665, 44.4255) -> (-85.9689, 57.708) centre (-87.9697, 51) ccw
  line L78 (-85.5665, 44.4255) -> (-90.7064, 35.6875)
  arc A71 (-95.6742, 27.2423) -> (-90.7064, 35.6875) centre (-97.5, 34) ccw
  line L79 (-95.6742, 27.2423) -> (-100.7064, 18.6875)
  arc A72 (-100.6571, 15.5255) -> (-100.7064, 18.6875) centre (-107.5, 17) ccw
  line L80 (-100.6571, 15.5255) -> (-95.5903, 6.7345)
  arc A73 (-104.2721, 1.7718) -> (-95.5903, 6.7345) centre (-97.5, 0) ccw
  line L81 (-104.2721, 1.7718) -> (-109.1246, 10.1911)
  arc A74 (-109.3258, 23.7577) -> (-109.1246, 10.1911) centre (-107.5, 17) ccw
  line L82 (-109.3258, 23.7577) -> (-104.2936, 32.3125)
  arc A75 (-104.3013, 35.6561) -> (-104.2936, 32.3125) centre (-97.5, 34) ccw
  line L83 (-104.3013, 35.6561) -> (-109.2417, 44.228)
  arc A76 (-108.7531, 57.8813) -> (-109.2417, 44.228) centre (-107.4697, 51) ccw
  line L84 (-108.7531, 57.8813) -> (-104.127, 65.7456)
  arc A77 (-104.329, 69.5378) -> (-104.127, 65.7456) centre (-97.5, 68) ccw
  line L85 (-104.329, 69.5378) -> (-109.3554, 78.2588)
  arc A78 (-100.6914, 83.2523) -> (-109.3554, 78.2588) centre (-107.4697, 85) ccw
  line L86 (-258.399, -5) -> (-268.101, -5)
  arc A79 (-275.8077, 6.4122) -> (-268.101, -5) centre (-273, 0) ccw
  line L87 (-275.8077, 6.4122) -> (-270.3189, 15.4181)
  arc A80 (-270.2059, 19.0076) -> (-270.3189, 15.4181) centre (-263.5, 17) ccw
  line L88 (-270.2059, 19.0076) -> (-274.9765, 27.2848)
  arc A81 (-274.8258, 40.7577) -> (-274.9765, 27.2848) centre (-273, 34) ccw
  line L89 (-274.8258, 40.7577) -> (-270.1078, 48.7783)
  arc A82 (-258.5707, 56) -> (-270.1078, 48.7783) centre (-263.4697, 51) ccw
  line L90 (-258.5707, 56) -> (-248.8686, 56)
  arc A83 (-241.5665, 44.4255) -> (-248.8686, 56) centre (-243.9697, 51) ccw
  line L91 (-241.5665, 44.4255) -> (-246.7064, 35.6875)
  arc A84 (-251.6742, 27.2423) -> (-246.7064, 35.6875) centre (-253.5, 34) ccw
  line L92 (-251.6742, 27.2423) -> (-256.7064, 18.6875)
  arc A85 (-256.6571, 15.5255) -> (-256.7064, 18.6875) centre (-263.5, 17) ccw
  line L93 (-256.6571, 15.5255) -> (-251.5903, 6.7345)
  arc A86 (-258.399, -5) -> (-251.5903, 6.7345) centre (-253.5, 0) ccw
  line L94 (-139.6914, 83.2523) -> (-134.8168, 74.7946)
  arc A87 (-134.0581, 61.4397) -> (-134.8168, 74.7946) centre (-136.5, 68) ccw
  line L95 (-134.0581, 61.4397) -> (-139.5557, 52.0938)
  arc A88 (-139.6625, 49.3685) -> (-139.5557, 52.0938) centre (-146.4697, 51) ccw
  line L96 (-139.6625, 49.3685) -> (-134.7042, 40.7657)
  arc A89 (-134.6742, 27.2423) -> (-134.7042, 40.7657) centre (-136.5, 34) ccw
  line L97 (-134.6742, 27.2423) -> (-139.7064, 18.6875)
  arc A90 (-144.6451, 10.2502) -> (-139.7064, 18.6875) centre (-146.5, 17) ccw
  line L98 (-144.6451, 10.2502) -> (-149.3471, 2.177)
  arc A91 (-158.8077, 6.4122) -> (-149.3471, 2.177) centre (-156, 0) ccw
  line L99 (-158.8077, 6.4122) -> (-153.3189, 15.4181)
  arc A92 (-153.2059, 19.0076) -> (-153.3189, 15.4181) centre (-146.5, 17) ccw
  line L100 (-153.2059, 19.0076) -> (-157.9765, 27.2848)
  arc A93 (-157.8258, 40.7577) -> (-157.9765, 27.2848) centre (-156, 34) ccw
  line L101 (-157.8258, 40.7577) -> (-153.1078, 48.7783)
  arc A94 (-147.7531, 57.8813) -> (-153.1078, 48.7783) centre (-146.4697, 51) ccw
  line L102 (-147.7531, 57.8813) -> (-143.127, 65.7456)
  arc A95 (-143.329, 69.5378) -> (-143.127, 65.7456) centre (-136.5, 68) ccw
  line L103 (-143.329, 69.5378) -> (-148.3554, 78.2588)
  arc A96 (-139.6914, 83.2523) -> (-148.3554, 78.2588) centre (-146.4697, 85) ccw
  line L104 (-285.7456, 32.1622) -> (-280.8454, 23.6602)
  arc A97 (-281.1451, 10.2502) -> (-280.8454, 23.6602) centre (-283, 17) ccw
  line L105 (-281.1451, 10.2502) -> (-285.8471, 2.177)
  arc A98 (-299.2721, 1.7718) -> (-285.8471, 2.177) centre (-292.5, 0) ccw
  line L106 (-299.2721, 1.7718) -> (-304.1246, 10.1911)
  arc A99 (-309.2059, 19.0076) -> (-304.1246, 10.1911) centre (-302.5, 17) ccw
  line L107 (-309.2059, 19.0076) -> (-313.9765, 27.2848)
  arc A100 (-313.8258, 40.7577) -> (-313.9765, 27.2848) centre (-312, 34) ccw
  line L108 (-313.8258, 40.7577) -> (-309.1078, 48.7783)
  arc A101 (-297.5707, 56) -> (-309.1078, 48.7783) centre (-302.4697, 51) ccw
  line L109 (-297.5707, 56) -> (-287.8686, 56)
  arc A102 (-280.5665, 44.4255) -> (-287.8686, 56) centre (-282.9697, 51) ccw
  line L110 (-280.5665, 44.4255) -> (-285.7064, 35.6875)
  arc A103 (-285.7456, 32.1622) -> (-285.7064, 35.6875) centre (-292.5, 34) ccw
  line L111 (-178.3077, 6.4122) -> (-172.8189, 15.4181)
  arc A104 (-172.7059, 19.0076) -> (-172.8189, 15.4181) centre (-166, 17) ccw
  line L112 (-172.7059, 19.0076) -> (-177.4765, 27.2848)
  arc A105 (-177.3258, 40.7577) -> (-177.4765, 27.2848) centre (-175.5, 34) ccw
  line L113 (-177.3258, 40.7577) -> (-172.6078, 48.7783)
  arc A106 (-172.7176, 52.8615) -> (-172.6078, 48.7783) centre (-165.9697, 51) ccw
  line L114 (-172.7176, 52.8615) -> (-177.5928, 61.3202)
  arc A107 (-176.7494, 74.8876) -> (-177.5928, 61.3202) centre (-175.5, 68) ccw
  line L115 (-176.7494, 74.8876) -> (-172.4118, 82.2615)
  arc A108 (-159.1914, 83.2523) -> (-172.4118, 82.2615) centre (-165.9697, 85) ccw
  line L116 (-159.1914, 83.2523) -> (-154.3168, 74.7946)
  arc A109 (-153.5581, 61.4397) -> (-154.3168, 74.7946) centre (-156, 68) ccw
  line L117 (-153.5581, 61.4397) -> (-159.0557, 52.0938)
  arc A110 (-163.5665, 44.4255) -> (-159.0557, 52.0938) centre (-165.9697, 51) ccw
  line L118 (-163.5665, 44.4255) -> (-168.7064, 35.6875)
  arc A111 (-168.7456, 32.1622) -> (-168.7064, 35.6875) centre (-175.5, 34) ccw
  line L119 (-168.7456, 32.1622) -> (-163.8454, 23.6602)
  arc A112 (-164.1451, 10.2502) -> (-163.8454, 23.6602) centre (-166, 17) ccw
  line L120 (-164.1451, 10.2502) -> (-168.8471, 2.177)
  arc A113 (-178.3077, 6.4122) -> (-168.8471, 2.177) centre (-175.5, 0) ccw
  line L121 (-120.1914, 83.2523) -> (-115.3168, 74.7946)
  arc A114 (-114.5581, 61.4397) -> (-115.3168, 74.7946) centre (-117, 68) ccw
  line L122 (-114.5581, 61.4397) -> (-120.0557, 52.0938)
  arc A115 (-120.1625, 49.3685) -> (-120.0557, 52.0938) centre (-126.9697, 51) ccw
  line L123 (-120.1625, 49.3685) -> (-115.2042, 40.7657)
  arc A116 (-115.1742, 27.2423) -> (-115.2042, 40.7657) centre (-117, 34) ccw
  line L124 (-115.1742, 27.2423) -> (-120.2064, 18.6875)
  arc A117 (-120.1571, 15.5255) -> (-120.2064, 18.6875) centre (-127, 17) ccw
  line L125 (-120.1571, 15.5255) -> (-115.0903, 6.7345)
  arc A118 (-121.899, -5) -> (-115.0903, 6.7345) centre (-117, 0) ccw
  line L126 (-121.899, -5) -> (-131.601, -5)
  arc A119 (-139.3077, 6.4122) -> (-131.601, -5) centre (-136.5, 0) ccw
  line L127 (-139.3077, 6.4122) -> (-133.8189, 15.4181)
  arc A120 (-128.8258, 23.7577) -> (-133.8189, 15.4181) centre (-127, 17) ccw
  line L128 (-128.8258, 23.7577) -> (-123.7936, 32.3125)
  arc A121 (-123.8013, 35.6561) -> (-123.7936, 32.3125) centre (-117, 34) ccw
  line L129 (-123.8013, 35.6561) -> (-128.7417, 44.228)
  arc A122 (-128.2531, 57.8813) -> (-128.7417, 44.228) centre (-126.9697, 51) ccw
  line L130 (-128.2531, 57.8813) -> (-123.627, 65.7456)
  arc A123 (-123.829, 69.5378) -> (-123.627, 65.7456) centre (-117, 68) ccw
  line L131 (-123.829, 69.5378) -> (-128.8554, 78.2588)
  arc A124 (-120.1914, 83.2523) -> (-128.8554, 78.2588) centre (-126.9697, 85) ccw
  line L132 (-217.6625, 49.3685) -> (-212.7042, 40.7657)
  arc A125 (-212.6742, 27.2423) -> (-212.7042, 40.7657) centre (-214.5, 34) ccw
  line L133 (-212.6742, 27.2423) -> (-217.7064, 18.6875)
  arc A126 (-217.6571, 15.5255) -> (-217.7064, 18.6875) centre (-224.5, 17) ccw
  line L134 (-217.6571, 15.5255) -> (-212.5903, 6.7345)
  arc A127 (-219.399, -5) -> (-212.5903, 6.7345) centre (-214.5, 0) ccw
  line L135 (-219.399, -5) -> (-229.101, -5)
  arc A128 (-240.7721, 1.7718) -> (-229.101, -5) centre (-234, 0) ccw
  line L136 (-240.7721, 1.7718) -> (-245.6246, 10.1911)
  arc A129 (-245.8258, 23.7577) -> (-245.6246, 10.1911) centre (-244, 17) ccw
  line L137 (-245.8258, 23.7577) -> (-240.7936, 32.3125)
  arc A130 (-235.8258, 40.7577) -> (-240.7936, 32.3125) centre (-234, 34) ccw
  line L138 (-235.8258, 40.7577) -> (-231.1078, 48.7783)
  arc A131 (-217.6625, 49.3685) -> (-231.1078, 48.7783) centre (-224.4697, 51) ccw
  line L139 (9.5303, 85) -> (-165.9697, 85) construction
  line L140 (20, 90) -> (-346, 90)
  line L141 (19.5, 0) -> (-351, 0) construction
  line L142 (-355, -5) -> (25, -5)
  line L143 (-195, 68) -> (-175.5, 68) construction
  line L144 (-196, 73) -> (-175, 73)
  line L145 (-321.9697, 51) -> (-204.9697, 51) construction
  line L146 (-322, 56) -> (-205, 56)
  dimension "d347" = 5
  dimension "d348" = 5
  dimension "d349" = 5
  dimension "d350" = 5
  constraint coincident A48.centre L139.start
  constraint coincident A108.centre L139.end
  constraint horizontal L140
  constraint coincident A42.centre L141.start
  constraint coincident A4.centre L141.end
  constraint horizontal L142
  constraint coincident A49.centre A57.centre
  constraint coincident A107.centre L143.end
  constraint parallel L143 L144
  constraint coincident A7.centre L145.start
  constraint coincident A56.centre L145.end
  constraint horizontal L146
  measures "d347" distance of L139 L140
  measures "d348" distance of L141 L142
  measures "d349" distance of L143 L144
  measures "d350" distance of L145 L146
extrude "Extrude17" cut sketch "Sketch8" against normal blind 2.2 contours L6 A0 L7 A1 L8 A2 A7 A98 L106 A99 L107 A100 L108 A101 L142 L146 | A83 L91 A84 L92 A85 L93 A86 A128 L136 A129 L137 A130 L138 A131 L142 L146 | A49 L56 A50 L57 A51 L58 A52 L59 A53 L111 A104 L112 A105 L113 A106 L114 A107 A113 L142 L144 | L94 A87 L95 A88 L96 A89 L97 A90 L98 A91 A96 A119 L127 A120 L128 A121 L129 A122 L130 A123 L131 A124 L140 L142 | A11 L18 A12 L19 A13 L20 A14 L21 A15 L22 A16 L76 A69 L77 A70 L78 A71 L79 A72 L80 A73 A78 L140 L142 | A22 L29 A23 L30 A24 L31 A25 L32 A26 L33 A27 A63 L71 A64 L72 A65 L73 A66 L74 A67 L75 A68 L140 L142 | L34 A28 L35 A29 L36 A30 L37 A31 L38 A32 A37 A43 L50 A44 L51 A45 L52 A46 L53 A47 L54 A48 L140 L142 bodies 1
extrude "Extrude18" add 1 faces at (2.2, 194.7842, 75.7727) along direction (-1, 0, 0) blind 2.2 on bodies 1 bodies 1
extrude "Extrude19" add 1 faces at (68.8, 194.7842, 75.7727) along direction (1, 0, 0) blind 2.2 on bodies 3 bodies 3
fillet "Fillet1" radius 7 2 edges at (6, 327.7275, 73.6318) (65, 327.7275, 73.6318) on bodies 1 3
fillet "Fillet1" radius 15 2 edges at (6, 348.4062, 44.7862) (65, 348.4062, 44.7862) on bodies 1 3
fillet "Fillet1" radius 2.5 2 edges at (6, 369, -12) (65, 369, -12) on bodies 1 3
fillet "Fillet1" radius 4 2 edges at (6, -31, 98) (65, -31, 98) on bodies 1 3
fillet "Fillet1" radius 4 2 edges at (6, -31, -12) (65, -31, -12) on bodies 1 3
extrude "Extrude20" cut sketch "Sketch7" against normal blind 3 contours A0 L142 L155 L156 | L142 L155 L156 L157 | L143 L155 L156 L157 | L3 L143 L155 L156 | L4 L152 L153 L154 | A38 L152 L153 L154 | A38 L140 L152 L153 bodies 3
extrude "Extrude21" cut sketch "Sketch7" against normal blind 13 contours L3 L143 L155 L156 | L4 L152 L153 L154 bodies 3
equation "d48 = ( 18 / 2 ) * 1 mm + 3 mm"
equation "d189 = ( 65 / 2 ) * 1 mm - 9 mm"
equation "paths = 5 mm"
equation "paristo = 18.5 mm"
equation "d252 = paristo"
equation "d290 = -paths"
equation "d322 = paths"
equation "d323 = -paths"
equation "d324 = paths"
equation "d325 = -paths"
